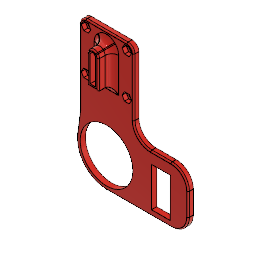
Mounting adapter 1 v7 (Autodesk Fusion 360 design; units mm, degrees)
Autodesk Fusion 360 part; units mm, degrees
note: some values were not read from the file. Set by a fixed rule: which sketch regions a step uses.
sketch "Sketch1" plane through (0, 38.5, 0) normal (0, 1, 0) x (-1, 0, 0)
  line L0 (2.0006, -20.791) -> (0.4096, -19.2)
  line L1 (0.4096, -19.2) -> (-0.4084, -19.2)
  line L2 (-0.4084, -19.2) -> (-1.9994, -20.791)
  line L3 (-1.9994, -20.791) -> (-1.9994, -40)
  line L4 (-1.9994, -40) -> (2.0006, -40)
  line L5 (2.0006, -40) -> (2.0006, -20.791)
  line L6 (-2.0094, -20.7869) -> (-2.0094, -40.01)
  line L7 (-2.0094, -40.01) -> (2.0106, -40.01)
  line L8 (2.0106, -40.01) -> (2.0106, -20.7869)
  line L9 (2.0106, -20.7869) -> (0.4138, -19.19)
  line L10 (0.4138, -19.19) -> (-0.4125, -19.19)
  line L11 (-0.4125, -19.19) -> (-2.0094, -20.7869)
  line L12 (-14.9994, -15.4248) -> (15.0006, -15.4248) construction
  line L13 (15.0006, -15.4248) -> (15.0006, -45.4248) construction
  line L14 (15.0006, -45.4248) -> (-14.9994, -45.4248) construction
  line L15 (-14.9994, -45.4248) -> (-14.9994, -15.4248) construction
  line L16 (-14.9994, -15.4248) -> (15.0006, -45.4248) construction
  line L17 (15.0006, -15.4248) -> (-14.9994, -45.4248) construction
  circle A0 centre (15.0006, -15.4248) radius 1.5
  circle A1 centre (-14.9994, -15.4248) radius 1.5
  circle A2 centre (15.0006, -45.4248) radius 1.5
  circle A3 centre (-14.9994, -45.4248) radius 1.5
  line L18 (20.0006, -10.4248) -> (20.0006, -50.4248)
  line L19 (20.0006, -50.4248) -> (-19.9994, -50.4248)
  line L20 (-19.9994, -50.4248) -> (-19.9994, -10.4248)
  line L21 (-19.9994, -10.4248) -> (20.0006, -10.4248)
  line L22 (-3.9994, -42) -> (4.0006, -42)
  line L23 (4.0006, -42) -> (4.0006, -19.9626)
  line L24 (4.0006, -19.9626) -> (1.238, -17.2)
  line L25 (1.238, -17.2) -> (-1.2368, -17.2)
  line L26 (-1.2368, -17.2) -> (-3.9994, -19.9626)
  line L27 (-3.9994, -19.9626) -> (-3.9994, -42)
  line L28 (13.2686, -12.4248) -> (11.5365, -15.4248)
  line L29 (11.5365, -15.4248) -> (13.2686, -18.4248)
  line L30 (13.2686, -18.4248) -> (16.7327, -18.4248)
  line L31 (16.7327, -18.4248) -> (18.4647, -15.4248)
  line L32 (18.4647, -15.4248) -> (16.7327, -12.4248)
  line L33 (16.7327, -12.4248) -> (13.2686, -12.4248)
  line L34 (-16.7314, -18.4248) -> (-13.2673, -18.4248)
  line L35 (-13.2673, -18.4248) -> (-11.5353, -15.4248)
  line L36 (-11.5353, -15.4248) -> (-13.2673, -12.4248)
  line L37 (-13.2673, -12.4248) -> (-16.7314, -12.4248)
  line L38 (-18.4635, -15.4248) -> (-16.7314, -18.4248)
  line L39 (-16.7314, -12.4248) -> (-18.4635, -15.4248)
  line L40 (13.2686, -48.4248) -> (16.7327, -48.4248)
  line L41 (16.7327, -48.4248) -> (18.4647, -45.4248)
  line L42 (18.4647, -45.4248) -> (16.7327, -42.4248)
  line L43 (16.7327, -42.4248) -> (13.2686, -42.4248)
  line L44 (11.5365, -45.4248) -> (13.2686, -48.4248)
  line L45 (13.2686, -42.4248) -> (11.5365, -45.4248)
  line L46 (-16.7314, -48.4248) -> (-13.2673, -48.4248)
  line L47 (-13.2673, -48.4248) -> (-11.5353, -45.4248)
  line L48 (-11.5353, -45.4248) -> (-13.2673, -42.4248)
  line L49 (-13.2673, -42.4248) -> (-16.7314, -42.4248)
  line L50 (-18.4635, -45.4248) -> (-16.7314, -48.4248)
  line L51 (-16.7314, -42.4248) -> (-18.4635, -45.4248)
  line L52 (20.0006, -50.4248) -> (-19.9994, -50.4248)
  line L53 (-19.9994, -50.4248) -> (-19.9994, -70.4248)
  line L54 (-19.9994, -70.4248) -> (20.0006, -70.4248)
  line L55 (20.0006, -70.4248) -> (20.0006, -50.4248)
  circle A4 centre (0.0006, -89.7248) radius 19.3
  circle A5 centre (0.0006, -89.7248) radius 22.3
  line L56 (-19.9994, -70.4248) -> (-22.117, -86.8782)
  line L57 (20.0006, -70.4248) -> (22.1182, -86.8782)
  line L58 (-19.9994, -50.4248) -> (0.0006, -50.4248)
  line L59 (0.0006, -50.4248) -> (0.0006, -112.0248)
  line L60 (0.0006, -112.0248) -> (-19.9994, -112.0248)
  line L61 (-19.9994, -112.0248) -> (-19.9994, -50.4248)
  line L62 (-19.9994, -112.0248) -> (-59.9994, -112.0248)
  line L63 (-59.9994, -112.0248) -> (-59.9994, -50.4248)
  line L64 (-59.9994, -50.4248) -> (-19.9994, -50.4248)
  line L65 (-19.9994, -50.4248) -> (-19.9994, -112.0248)
  line L66 (-33.0994, -78.8248) -> (-46.8994, -78.8248)
  line L67 (-46.8994, -78.8248) -> (-46.8994, -107.6248)
  line L68 (-46.8994, -107.6248) -> (-33.0994, -107.6248)
  line L69 (-33.0994, -107.6248) -> (-33.0994, -78.8248)
  line L70 (-33.0994, -78.8248) -> (-46.8994, -107.6248) construction
  line L71 (-46.8994, -78.8248) -> (-33.0994, -107.6248) construction
  line L72 (-19.9994, -50.4248) -> (-59.9994, -50.4248)
  line L73 (-59.9994, -50.4248) -> (-59.9994, -70.4248)
  line L74 (-59.9994, -70.4248) -> (-19.9994, -70.4248)
  line L75 (-19.9994, -70.4248) -> (-19.9994, -50.4248)
  point P0 (0.0006, -30.4248)
  point P1 (15.0006, -15.4248)
  point P2 (-39.9994, -93.2248)
  dimension "d254" = 0.01
  dimension "d255" = 30
  dimension "d256" = 30
  dimension "d257" = 3
  dimension "d260" = -30
  dimension "d261" = -30
  dimension "d262" = 5
  dimension "d263" = 2
  dimension "d323" = 3
  dimension "d326" = -30
  dimension "d327" = -30
  dimension "d1" = 20
  dimension "d2" = 38.6
  dimension "d3" = 3
  dimension "d4" = 40
  dimension "d5" = 28.8
  dimension "d6" = 13.8
  constraint perpendicular L12 L13
  constraint parallel L12 L14
  constraint parallel L13 L15
  constraint horizontal L12
  constraint coincident L16 P0
  constraint coincident L17 P0
  constraint coincident P1 L12.end
  constraint horizontal L52
  constraint vertical L53
  constraint horizontal L54
  constraint vertical L55
  constraint coincident A5 L56.end
  constraint tangent A5 L56
  constraint coincident A5 L57.end
  constraint tangent A5 L57
  constraint horizontal L58
  constraint vertical L59
  constraint horizontal L60
  constraint vertical L61
  constraint coincident A5 L59.end
  constraint horizontal L62
  constraint vertical L63
  constraint horizontal L64
  constraint vertical L65
  constraint perpendicular L66 L67
  constraint parallel L66 L68
  constraint parallel L67 L69
  constraint horizontal L66
  constraint coincident L70 P2
  constraint coincident L71 P2
  constraint horizontal L72
  constraint vertical L73
  constraint horizontal L74
  constraint vertical L75
  constraint coincident L63 L73.end
  measures "d255" distance of P1 L13.end
  measures "d256" distance of L13.end L14.end
  measures "d257" diameter of A0
  measures "d323" distance of P1 L33
  measures "d1" distance of L18.end L54.end
  measures "d2" diameter of A4
  measures "d4" distance of L60.end L62.end
  measures "d5" distance of L66.end L67.end
  measures "d6" distance of L67.end L68.end
extrude "Extrude2" add sketch "Sketch1" along normal blind 2 contours L0 L1 L2 L3 L4 L5 | L6 L7 L8 L9 L10 L11 | L18 L19 L20 L21 L52 L58 | L19 L52 L54 L55 A5 L59 | L19 L52 L53 L54 A5 L58 L59 L61 L65 L75 | L54 A5 L57 | L54 A5 L59 | L54 A5 L59 | L54 A4 A5 L59 | A5 L56 L61 L65 | L54 A5 L61 L65 | A5 L56 L61 L62 L63 L65 L74 | L54 A4 A5 L59 L61 L65 | A5 L61 L65 | A5 L60 L61 L65 | L22 L23 L24 L25 L26 L27 makes body 1
extrude "Extrude1" add sketch "Sketch1" against normal blind 10 contours L22 L23 L24 L25 L26 L27 bodies 1
fillet "Fillet2" radius 3.5 4 edges at (-1.238, 33.5, -17.2) (-4.0006, 33.5, -19.9626) (1.2368, 33.5, -17.2) (3.9994, 33.5, -19.9626) on bodies 1
fillet "Fillet3" radius 5 8 edges at (-4.0006, 38.5, -31.7062) (-3.7342, 38.5, -20.0729) (-2.7255, 38.5, -18.6874) (-0.0006, 38.5, -17.4123) (2.7243, 38.5, -18.6874) (3.733, 38.5, -20.0729) (3.9994, 38.5, -31.7062) (-0.0006, 38.5, -42) on bodies 1
extrude "Extrude3" add 1 faces at (-0.4814, 40.5, -55.7761) along direction (0, 1, 0) blind 1 on bodies 1 bodies 1
extrude "Extrude4" add sketch "Sketch1" along normal blind 3 and the other way blind -4 separate body contours L28 L29 L30 L31 L32 L33 | L34 L35 L36 L37 L38 L39 | L40 L41 L42 L43 L44 L45 | L46 L47 L48 L49 L50 L51 makes body 2 at (-15.038, 42.5, -17.9234) makes body 3 at (-12.8181, 42.5, -46.6417) makes body 4 at (17.1819, 42.5, -16.6417) makes body 5 at (17.1819, 42.5, -46.6417)
extrude "Extrude5" add 1 faces at (-0.4814, 41.5, -55.7761) along direction (0, 1, 0) blind 1 on bodies 1 bodies 1 2 3 4 5
extrude "Extrude6" cut sketch "Sketch1" along normal blind 2 contours L0 L1 L2 L3 L4 L5 bodies 1
extrude "Extrude7" cut sketch "Sketch1" along normal blind 2 contours L6 L7 L8 L9 L10 L11 bodies 1
fillet "Fillet7" radius 1 8 edges at (3.9994, 28.5, -31.7062) (3.733, 28.5, -20.0729) (2.7243, 28.5, -18.6874) (-0.0006, 28.5, -17.4123) (-2.7255, 28.5, -18.6874) (-3.7342, 28.5, -20.0729) (-4.0006, 28.5, -31.7062) (-0.0006, 28.5, -42) on bodies 1
fillet "Fillet11" radius 12.5 3 edges at (19.9994, 40.5, -70.4248) (59.9994, 40.5, -70.4248) (59.9994, 40.5, -112.0248) on bodies 1
fillet "Fillet12" radius 5 2 edges at (19.9994, 40.5, -10.4248) (-20.0006, 40.5, -10.4248) on bodies 1
fillet "Fillet13" radius 1 13 edges at (-21.0594, 38.5, -78.6515) (-20.0006, 38.5, -42.9248) (-18.5362, 38.5, -11.8893) (-0.0006, 38.5, -10.4248) (18.5349, 38.5, -11.8893) (19.9994, 38.5, -36.6748) (23.6605, 38.5, -66.7636) (39.9994, 38.5, -70.4248) (56.3382, 38.5, -74.086) (59.9994, 38.5, -91.2248) (56.3382, 38.5, -108.3636) (23.7494, 38.5, -112.0248) (-16.7453, 38.5, -104.4525) on bodies 1
